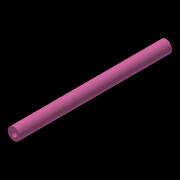
# Autodesk Inventor part: Long Pool Noodle
Saved by Autodesk Inventor 2014 SP1 (Build 180222100, 222)
## iProperties
Created: 2013-11-30
Part Number: Long Pool Noodle
Material: Generic
Document SubType Name: Modeling
Designer: Rauhul Varma
Mass: 1972.64 g
Surface Area: 2309.79 cm^2
Volume: 1972.64 cm^3
Density: 1 g/cm^3
Appearance: Pink
Author: Rauhul Varma
Autodesk Inventor part; units mm, degrees
ref_plane "YZ Plane" through (0, 0, 0) normal (1, 0, 0) x (0, 1, 0)
ref_plane "XZ Plane" through (0, 0, 0) normal (0, 1, 0) x (-1, 0, 0)
ref_plane "XY Plane" through (0, 0, 0) normal (0, 0, 1) x (1, 0, 0)
sketch "Sketch1" plane through (0, 0, 0) normal (0, 0, 1) x (1, 0, 0)
  circle A0 centre (0, 0) radius 31.75
  circle A1 centre (0, 0) radius 14.2875
  dimension "d0" = 63.5
  dimension "d1" = 28.575
  constraints: 2 centre point, 2 coincident
  measures "d0" diameter of A0
  measures "d1" diameter of A1
extrude "Extrusion1" add sketch "Sketch1" along normal blind 781.05
body "Solid1"
